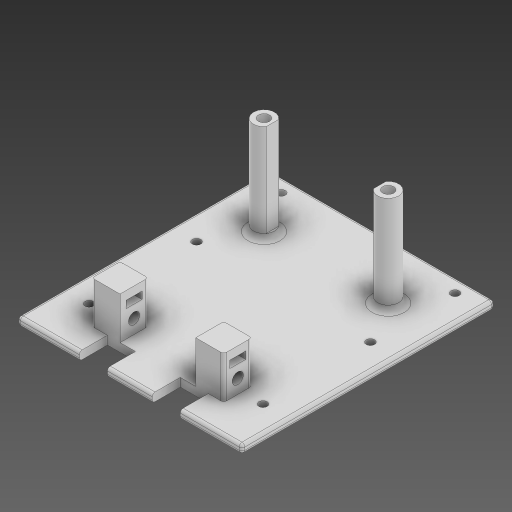
# Autodesk Inventor part: kreplenie_dribler_V4
Saved by Autodesk Inventor 2023 (Build 270158000, 158)
## iProperties
Created: 2025-07-15
Part Number: kreplenie_dribler_V4
Material: Типовые
Document SubType Name: Modeling
Designer: daa
Density: 1 g/cm^3
Appearance: По умолчанию
Author: daa
Autodesk Inventor part; units mm, degrees
ref_plane "YZ Plane" through (0, 0, 0) normal (1, 0, 0) x (0, 1, 0)
ref_plane "XZ Plane" through (0, 0, 0) normal (0, 1, 0) x (-1, 0, 0)
ref_plane "XY Plane" through (0, 0, 0) normal (0, 0, 1) x (1, 0, 0)
sketch "Эскиз1" plane through (0, 0, 0) normal (0, 1, 0) x (-1, 0, 0)
  line L0 (6, 63) -> (-74, 63)
  line L1 (-74, 63) -> (-74, -27)
  line L2 (-74, -27) -> (6, -27)
  line L3 (6, -27) -> (6, 63)
  line L4 (-3, 8.202) -> (-65, 8.202)
  line L5 (-65, 8.202) -> (-65, -22)
  line L6 (-65, -22) -> (-3, -22)
  line L7 (-3, -22) -> (-3, 8.202)
  circle A0 centre (-3, 8.202) radius 1.5
  circle A1 centre (-3, -22) radius 1.5
  circle A2 centre (-65, 8.202) radius 1.5
  circle A3 centre (-65, -22) radius 1.5
  circle A4 centre (-3, 46.5) radius 1.5
  circle A5 centre (-65, 46.5) radius 1.5
  point P0 (0, 0)
  dimension "d0" = 80
  dimension "d1" = 90
  dimension "d2" = 30.202
  dimension "d3" = 5
  dimension "d4" = 62
  dimension "d5" = 9
  dimension "d6" = 3
  dimension "d7" = 3
  dimension "d8" = 3
  dimension "d9" = 3
  dimension "d10" = 3
  dimension "d11" = 9
  dimension "d12" = 16.5
  dimension "d13" = 3
  dimension "d14" = 16.5
  dimension "d15" = 9
  constraints: 16 end point, 6 centre point, 4 coincident, 4 parallel, 2 horizontal, 2 perpendicular
  measures "d0" distance of L2.end L1.end
  measures "d1" distance of L1.end L0.end
  measures "d2" distance of L6.end L4.start
  measures "d3" distance between parallel lines of L2 L6
  measures "d4" distance of L4.start L4.end
  measures "d5" distance between parallel lines of L3 L7
  measures "d6" diameter of A0
  measures "d7" diameter of A1
  measures "d8" diameter of A2
  measures "d9" diameter of A3
  measures "d10" diameter of A4
  measures "d11" distance from line of L3 A4.centre
  measures "d12" distance from line of A4.centre L0
  measures "d13" diameter of A5
  measures "d14" distance from line of A5.centre L0
  measures "d15" distance from line of L1 A5.centre
extrude "Выдавливание1" add sketch "Эскиз1" along normal blind 3 contours L3 L2 L1 L0 | L4 A0 L7 A1 L6 A3 L5 A2
sketch "Эскиз2" plane through (0, 3, 0) normal (0, 1, 0) x (1, 0, 0)
  line L0 (10.5, -53) -> (20.5, -53)
  line L1 (20.5, -53) -> (20.5, -43)
  line L2 (20.5, -43) -> (10.5, -43)
  line L3 (10.5, -43) -> (10.5, -53)
  line L4 (47.5, -53) -> (57.5, -53)
  line L5 (57.5, -53) -> (57.5, -43)
  line L6 (57.5, -43) -> (47.5, -43)
  line L7 (47.5, -43) -> (47.5, -53)
  line L8 (-6, -63) -> (74, -63) projected
  line L9 (-6, 27) -> (-6, -63) projected
  point P0 (0, 0)
  point P1 (15.5, -53)
  point P2 (20.5, -48)
  dimension "d18" = 10
  dimension "d19" = 10
  dimension "d20" = 10
  dimension "d21" = 27
  dimension "d23" = 10
  dimension "d24" = 16.5
  constraints: 16 end point, 4 parallel, 2 horizontal, 2 midpoint, 2 perpendicular, 2 point on line
  measures "d18" distance from line of point (15.5, -53) L8
  measures "d19" distance of L2.end L0.start
  measures "d20" distance of L1.end L2.end
  measures "d21" distance from line of L7 point (20.5, -48)
  measures "d23" distance of L5.end L6.end
  measures "d24" distance from line of L9 L2.end
extrude "Выдавливание2" add sketch "Эскиз2" along normal blind 15
sketch "Эскиз3" plane through (57.5, 3, 53) normal (1, 0, 0) x (0, 0, -1)
  line L0 (2.15, 12) -> (7.85, 12)
  line L1 (7.85, 12) -> (7.85, 9.4)
  line L2 (7.85, 9.4) -> (2.15, 9.4)
  line L3 (2.15, 9.4) -> (2.15, 12)
  circle A0 centre (5, 5) radius 2
  line L4 (0, 15) -> (10, 15) projected
  line L5 (10, 0) -> (10, 15) projected
  point P0 (53, -3)
  dimension "d27" = 4
  dimension "d28" = 5.7
  dimension "d29" = 2.6
  dimension "d30" = 3
  dimension "d31" = 2.15
  dimension "d32" = 10
  dimension "d33" = 5
  constraints: 8 end point, 2 parallel, 1 centre point, 1 horizontal, 1 perpendicular
  measures "d27" diameter of A0
  measures "d28" distance of L1.end L2.end
  measures "d29" distance of L0.end L1.end
  measures "d30" distance between parallel lines of L4 L0
  measures "d31" distance between parallel lines of L5 L1
  measures "d32" distance from line of L4 A0.centre
  measures "d33" distance from line of L5 A0.centre
extrude "Выдавливание3" cut sketch "Эскиз3" against normal blind 78
fillet "Сопряжение2" radius 1 12 edges at (74, 0, 18) (74, 3, 18) (34, 0, -27) (74, 1.5, -27) (34, 3, -27) (-6, 3, 18) (-6, 0, 18) (34, 3, 63) (34, 0, 63) (-6, 1.5, 63) (74, 1.5, 63) (-6, 1.5, -27)
sketch "Эскиз6" plane through (0, 3, 0) normal (0, 1, 0) x (1, 0, 0)
  line L0 (14, 16) -> (-1, 16)
  line L1 (-1, 16) -> (-1, -2)
  line L2 (-1, -2) -> (14, -2)
  line L3 (14, -2) -> (14, 16)
  line L4 (73, 27) -> (-5, 27) projected
  line L5 (-6, 26) -> (-6, -62) projected
  line L6 (69, 16) -> (54, 16)
  line L7 (54, 16) -> (54, -2)
  line L8 (54, -2) -> (69, -2)
  line L9 (69, -2) -> (69, 16)
  line L10 (74, -62) -> (74, 26) projected
  circle A0 centre (11.85, 7) radius 2
  circle A1 centre (11.85, 7) radius 3.75
  circle A2 centre (56.15, 7) radius 2
  circle A3 centre (56.15, 7) radius 3.75
  point P0 (0, 0)
  dimension "d38" = 15
  dimension "d39" = 18
  dimension "d40" = 11
  dimension "d41" = 5
  dimension "d42" = 15
  dimension "d43" = 18
  dimension "d44" = 11
  dimension "d45" = 5
  dimension "d49" = 4
  dimension "d50" = 7.5
  dimension "d51" = 4
  dimension "d52" = 7.5
  dimension "d54" = 44.3
  dimension "d56" = 17.85
  constraints: 16 end point, 4 centre point, 4 parallel, 2 coincident, 2 horizontal, 2 perpendicular
  measures "d38" distance of L2.end L1.end
  measures "d39" distance of L1.end L0.end
  measures "d40" distance from line of L0.end L4
  measures "d41" distance between parallel lines of L5 L1
  measures "d42" distance of L8.end L7.end
  measures "d43" distance of L7.end L6.end
  measures "d44" distance between parallel lines of L6 L4
  measures "d45" distance between parallel lines of L10 L9
  measures "d49" diameter of A0
  measures "d50" diameter of A1
  measures "d51" diameter of A2
  measures "d52" diameter of A3
  measures "d54" distance of A2.centre A0.centre
  measures "d56" distance from line of L10 A2.centre
extrude "Выдавливание4" add sketch "Эскиз6" along normal blind 35 contours A1 L3 | L3 A1 | A3 L7 | L7 A3
fillet "Сопряжение4" radius 2 2 edges at (8.1, 3, -7) (52.4, 3, -7)
sketch "Эскиз7" plane through (11.85, 38, -7) normal (0, 1, 0) x (1, 0, 0)
  circle A0 centre (0, 0) radius 3.75 projected
  line L0 (3, 2.25) -> (3, -2.25)
  circle A1 centre (44.3, 0) radius 3.75 projected
  line L1 (41.3, 2.25) -> (41.3, -2.25)
  point P0 (-11.85, -7)
  constraints: 4 end point, 4 point on circle, 2 vertical
extrude "Выдавливание5" cut sketch "Эскиз7" against normal blind 33 contours A0 L0 | L1 A1 picked at (3.1367, -0.52) picked at (41.1633, -0.52)
fillet "Сопряжение5" radius 1 6 edges at (10.5, 10.5, 43) (20.5, 10.5, 43) (47.5, 10.5, 43) (57.5, 10.5, 43) (57.5, 10.5, 53) (10.5, 10.5, 53)
sketch "Эскиз12" plane through (0, 3, 0) normal (0, 1, 0) x (1, 0, 0)
  line L0 (73, -63) -> (-5, -63) projected
  line L1 (11.5, -53) -> (20.5, -53) projected
  line L2 (16, -53) -> (26, -53)
  line L3 (26, -53) -> (26, -63)
  line L4 (26, -63) -> (16, -63)
  line L5 (16, -63) -> (16, -53)
  line L6 (47.5, -53) -> (56.5, -53) projected
  line L7 (52, -53) -> (42, -53)
  line L8 (42, -53) -> (42, -63)
  line L9 (42, -63) -> (52, -63)
  line L10 (52, -63) -> (52, -53)
  point P0 (0, 0)
  constraints: 16 end point, 4 parallel, 2 horizontal, 2 midpoint, 2 perpendicular, 2 point on line
extrude "Выдавливание9" cut sketch "Эскиз12" against normal blind 10
